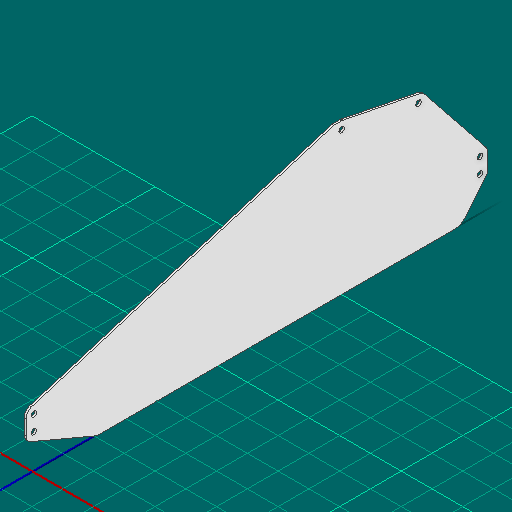
# Autodesk Inventor part: skirt
Saved by Autodesk Inventor 2025 (Build 290162000, 162)
## iProperties
Created: 2024-09-29
Part Number: skirt
Material: Acetal Resin, White
Document SubType Name: Modeling
Designer: averey
Density: 1.425 g/cm^3
Appearance: Smooth - White
Author: averey
Autodesk Inventor part; units mm, degrees
ref_plane "YZ Plane" through (0, 0, 0) normal (1, 0, 0) x (0, 1, 0)
ref_plane "XZ Plane" through (0, 0, 0) normal (0, 1, 0) x (-1, 0, 0)
ref_plane "XY Plane" through (0, 0, 0) normal (0, 0, 1) x (1, 0, 0)
sketch "maiin" plane through (0, 0, 0) normal (0, 0, 1) x (1, 0, 0)
  circle A0 centre (114.3234, 350.4213) radius 2.1844
  circle A1 centre (127.0234, 350.4213) radius 2.1844
  line L0 (86.4201, 300.7833) -> (108.4755, 352.8962)
  arc A2 (86.4201, 300.7833) -> (85.4157, 295.8335) centre (98.1157, 295.8335) ccw
  line L1 (209.5734, 102.7713) -> (133.0946, 352.2822)
  line L2 (209.5734, 96.4213) -> (209.5734, 102.7713)
  circle A3 centre (203.2234, 96.4213) radius 2.1844
  arc A4 (209.45, 95.176) -> (209.5734, 96.4213) centre (203.2234, 96.4213) ccw
  line L3 (196.75, 31.676) -> (209.45, 95.176)
  circle A5 centre (190.5234, 32.9213) radius 2.1844
  line L4 (85.4157, 295.8335) -> (85.4157, 3.6912)
  circle A6 centre (127.0234, -17.8787) radius 2.1844
  circle A7 centre (114.3234, -17.8787) radius 2.1844
  arc A8 (127.0234, -24.2287) -> (130.9902, -22.8372) centre (127.0234, -17.8787) ccw
  arc A9 (110.2871, -22.7809) -> (114.3234, -24.2287) centre (114.3234, -17.8787) ccw
  arc A10 (194.4902, 27.9628) -> (196.75, 31.676) centre (190.5234, 32.9213) ccw
  arc A11 (85.4157, 3.6912) -> (90.0433, -6.1132) centre (98.1157, 3.6912) ccw
  line L5 (130.9902, -22.8372) -> (194.4902, 27.9628)
  line L6 (110.2871, -22.7809) -> (90.0433, -6.1132)
  line L7 (114.3234, -24.2287) -> (127.0234, -24.2287)
  arc A12 (114.3234, 356.7713) -> (108.4755, 352.8962) centre (114.3234, 350.4213) ccw
  line L8 (127.0234, 356.7713) -> (114.3234, 356.7713)
  arc A13 (133.0946, 352.2822) -> (127.0234, 356.7713) centre (127.0234, 350.4213) ccw
  point P0 (137.6055, 139.9011)
  point P1 (110.8157, 355.7146)
  dimension "d0" = 12.7
  dimension "d1" = 12.7
  dimension "d2" = 25.4
  measures "d0" diameter of A4
  measures "d1" radius of A11
  measures "d2" distance from line of point (110.816, 355.715) L4
sketch "Sketch1" plane through (0, 0, 0) normal (1, 0, 0) x (0, 1, 0)
  circle A0 centre (-12.7, 0) radius 2.1844
  circle A1 centre (0, 0) radius 2.1844
  line L0 (-40.6033, -49.6379) -> (-18.5478, 2.4749)
  arc A2 (-40.6033, -49.6379) -> (-41.6076, -54.5878) centre (-28.9076, -54.5878) ccw
  line L1 (82.55, -247.65) -> (6.0712, 1.8609)
  line L2 (82.55, -254) -> (82.55, -247.65)
  circle A3 centre (76.2, -254) radius 2.1844
  arc A4 (82.4267, -255.2453) -> (82.55, -254) centre (76.2, -254) ccw
  line L3 (69.7267, -318.7453) -> (82.4267, -255.2453)
  circle A5 centre (63.5, -317.5) radius 2.1844
  line L4 (-41.6076, -54.5878) -> (-41.6076, -346.7301)
  circle A6 centre (0, -368.3) radius 2.1844
  circle A7 centre (-12.7, -368.3) radius 2.1844
  arc A8 (0, -374.65) -> (3.9668, -373.2585) centre (0, -368.3) ccw
  arc A9 (-16.7362, -373.2022) -> (-12.7, -374.65) centre (-12.7, -368.3) ccw
  arc A10 (67.4668, -322.4585) -> (69.7267, -318.7453) centre (63.5, -317.5) ccw
  arc A11 (-41.6076, -346.7301) -> (-36.98, -356.5344) centre (-28.9076, -346.7301) ccw
  line L5 (3.9668, -373.2585) -> (67.4668, -322.4585)
  line L6 (-16.7362, -373.2022) -> (-36.98, -356.5344)
  line L7 (-12.7, -374.65) -> (0, -374.65)
  arc A12 (-12.7, 6.35) -> (-18.5478, 2.4749) centre (-12.7, 0) ccw
  line L8 (0, 6.35) -> (-12.7, 6.35)
  arc A13 (6.0712, 1.8609) -> (0, 6.35) centre (0, 0) ccw
  constraints: 1 other
extrude "Extrusion1" add sketch "Sketch1" along normal blind 1.5875
body "Solid1"
